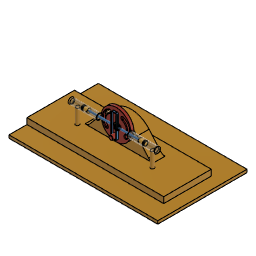
Scotch Yoke Mechanism FINISHED (Autodesk Fusion 360 design; units mm, degrees)
Autodesk Fusion 360 part; units mm, degrees
sketch "Bottom Sketch" plane through (0, 0, 0) normal (0, 0, 1) x (1, 0, 0) in component "Holder"
  line L0 (0, 0) -> (250, 0)
  line L1 (250, 0) -> (250, 150)
  line L2 (250, 150) -> (0, 150)
  line L3 (0, 150) -> (0, 0)
  dimension "d1" = 250
  dimension "d2" = 150
  constraint horizontal L0
  constraint vertical L1
  constraint horizontal L2
  constraint vertical L3
  constraint coincident L0.start L3.end
  measures "d1" distance of L0.start L0.end
  measures "d2" distance of L0.start L2.end
extrude "Extrude1" add sketch "Bottom Sketch" along normal blind 5 makes body 1 in component "Holder"
sketch "holder" plane through (0, 0, 5) normal (0, 0, 1) x (-1, 0, 0) in component "Holder"
  line L0 (0, -150) -> (0, 0)
  line L1 (0, 0) -> (-250, 0)
  line L2 (-250, 0) -> (-250, -150)
  line L3 (-250, -150) -> (0, -150)
  circle A0 centre (-205.8519, -60.5247) radius 10
  line L4 (0, -150) -> (-125, -150)
  line L5 (-125, -150) -> (-125, 0)
  circle A1 centre (-44.1481, -60.5247) radius 10
  dimension "d5" = 20
  dimension "d6" = 125
  constraint coincident L0.start L3.end
  constraint midpoint L3 L4.end
  constraint midpoint L1 L5.end
  constraint symmetric A0 L5 A1
  measures "d5" diameter of A0
  measures "d6" distance of L0.start L4.end
extrude "Extrude2" add sketch "holder" along normal blind 10 separate body contours A0 makes body 2 in component "Holder"
extrude "Extrude3" add sketch "holder" along normal blind 10 contours A1 bodies 1 in component "Holder"
combine "Combine1" operation add target body 1 tool bodies 2 in component "Holder"
sketch "holder nr2" plane through (0, 0, 15) normal (0, 0, 1) x (-1, 0, 0) in component "Holder"
  circle A0 centre (-205.8519, -60.5247) radius 10
  line L0 (-240, -20) -> (-10, -20)
  line L1 (-10, -20) -> (-10, -100)
  line L2 (-10, -100) -> (-240, -100)
  line L3 (-240, -100) -> (-240, -20)
  constraint horizontal L0
  constraint vertical L1
  constraint horizontal L2
  constraint vertical L3
extrude "Extrude4" add sketch "holder nr2" along normal blind 10 contours A0 | L0 L1 L2 L3 bodies 1 in component "Holder"
sketch "holder circle" plane through (0, 100, 0) normal (0, 1, 0) x (-1, 0, 0) in component "Holder"
  line L0 (-240, 15) -> (-10, 15)
  line L1 (-10, 15) -> (-10, 25)
  line L2 (-10, 25) -> (-240, 25)
  line L3 (-240, 25) -> (-240, 15)
  line L4 (-177.5741, 25) -> (-155.4332, 50.958)
  line L5 (-125, 65) -> (-125, 15)
  line L6 (-72.4259, 25) -> (-94.5668, 50.958)
  arc A0 (-94.5668, 50.958) -> (-155.4332, 50.958) centre (-125, 25) ccw
  constraint coincident L2 L4.start
  constraint midpoint L0 L5.end
  constraint symmetric L4.start L5 L6.start
  constraint symmetric L4.end L5 L6.end
extrude "Extrude5" add sketch "holder circle" along normal blind -20 and the other way blind 40 contours L2 L5 L6 A0 | L2 L4 L5 A0 bodies 1 in component "Holder"
sketch "crank" plane through (0, 0, 0) normal (0, 1, 0) x (1, 0, 0) in component "Crank"
  circle A0 centre (125, -55) radius 25
  circle A1 centre (125, -55) radius 3
  circle A2 centre (125, -40) radius 3.5
  dimension "d18" = 50
  dimension "d19" = 6
  dimension "d24" = 7
  constraint concentric A0 A1
  measures "d18" diameter of A0
  measures "d19" diameter of A1
  measures "d24" diameter of A2
extrude "Extrude1'" add sketch "crank" along normal blind 60 and the other way blind -55 separate body contours A0 | A2 makes body 3 in component "Crank"
extrude "Extrude2'" add sketch "crank" along normal blind 60 and the other way blind -46 contours A2 bodies 3 in component "Crank"
fillet "Fillet1" radius 0.5 1 faces at (123.924, 46, 39.8261) on bodies 3 in component "Crank"
sketch "crank holder" plane through (0, 60, 0) normal (0, -1, 0) x (1, 0, 0) in component "Holder"
  line L0 (94.5668, 50.958) -> (72.4259, 25)
  line L1 (72.4259, 25) -> (177.5741, 25)
  line L2 (177.5741, 25) -> (155.4332, 50.958)
  arc A0 (155.4332, 50.958) -> (94.5668, 50.958) centre (125, 25) ccw
  circle A1 centre (125, 55) radius 2.996
extrude "Extrude6" add sketch "crank holder" along normal blind 6 contours A1 bodies 1 in component "Holder"
fillet "Fillet1'" radius 0.25 1 edges at (122.2068, 54, 53.9166) on bodies 1 in component "Holder"
sketch "crank button" plane through (0, 54, 0) normal (0, -1, 0) x (1, 0, 0) in component "Holder"
  circle A0 centre (125, 55) radius 2.746
  circle A1 centre (125, 55) radius 1.0708
  constraint concentric A0 A1
extrude "Extrude7" add sketch "crank button" along normal blind 0.5 contours A1 bodies 1 in component "Holder"
fillet "Fillet2" radius 0.5 1 edges at (124.0017, 53.5, 54.6128) on bodies 1 in component "Holder"
sketch "crank design" plane through (0, 55, 0) normal (0, -1, 0) x (1, 0, 0) in component "Crank"
  circle A0 centre (125, 40) radius 3.5
  circle A1 centre (125, 55) radius 3
  circle A2 centre (125, 55) radius 25
  line L0 (125, 58) -> (125, 30)
  arc A3 (139.6103, 45.9052) -> (135.2122, 67.1617) centre (130, 55) ccw
  arc A4 (142.5156, 43.1557) -> (136.7878, 70.8383) centre (130, 55) ccw
  arc A5 (113.2122, 70.8383) -> (107.4844, 43.1557) centre (120, 55) ccw
  arc A6 (114.7878, 67.1617) -> (110.3897, 45.9052) centre (120, 55) ccw
  arc A7 (136.7878, 70.8383) -> (135.2122, 67.1617) centre (136, 69) ccw
  arc A8 (139.6103, 45.9052) -> (142.5156, 43.1557) centre (141.0629, 44.5304) ccw
  arc A9 (107.4844, 43.1557) -> (110.3897, 45.9052) centre (108.9371, 44.5304) ccw
  arc A10 (114.7878, 67.1617) -> (113.2122, 70.8383) centre (114, 69) ccw
  constraint coincident A2 L0.end
  constraint vertical L0
  constraint symmetric L0 A7 A10
  constraint symmetric L0 A8 A9
  constraint symmetric L0 A4.end A5.start
  constraint symmetric L0 A3.end A6.start
  constraint symmetric L0 A3.start A6.end
  constraint symmetric L0 A3 A6
  constraint symmetric L0 A4 A5
  constraint symmetric L0 A4.start A5.end
  constraint coincident A1 L0.start
extrude "Extrude3'" cut sketch "crank design" against normal blind 5 contours A3 A4 A7 A8 | A5 A6 A9 A10 bodies 3 in component "Crank"
fillet "Fillet2'" radius 1 tangency weight 1.30642 8 edges at (139.6882, 55, 43.0778) (142.9571, 55, 57.6809) (134.1617, 55, 69.7878) (146.8741, 55, 58.4914) (115.8383, 55, 69.7878) (107.0429, 55, 57.6809) (110.3118, 55, 43.0778) (103.1259, 55, 58.4914) on bodies 3 in component "Crank"
fillet "Fillet3" radius 1 8 edges at (142.9571, 60, 57.6809) (139.6882, 60, 43.0778) (146.8741, 60, 58.4914) (134.1617, 60, 69.7878) (110.3118, 60, 43.0778) (107.0429, 60, 57.6809) (115.8383, 60, 69.7878) (103.1259, 60, 58.4914) on bodies 3 in component "Crank"
fillet "Fillet3'" radius 10 2 edges at (72.4259, 70, 25) (177.5741, 70, 25) on bodies 1 in component "Holder"
sketch "slider part" plane through (0, 55, 0) normal (0, -1, 0) x (1, 0, 0) in component "Slider"
  spline S0 degree 3 poles (138.884, 46.5925) (138.6466, 46.3416) (138.4537, 46.0504) (138.0969, 45.2368) (138.0174, 44.6763) (138.144, 43.7208) (138.2876, 43.3168) (138.644, 42.7368) (138.8105, 42.5316) (139.0008, 42.3515) (139.2187, 42.1453) (139.4677, 41.9721) (140.1668, 41.6275) (140.6495, 41.5207) (141.7193, 41.5441) (142.3066, 41.7372) (142.9525, 42.1918) (143.1044, 42.3231) (143.2419, 42.4684) knots -0.939789 -0.939789 -0.939789 -0.939789 -0.836626 -0.836626 -0.673634 -0.673634 -0.548256 -0.548256 -0.469895 -0.469895 -0.469895 -0.380181 -0.380181 -0.236639 -0.236639 -0.059698 -0.059698 0 0 0 0
  spline S1 degree 3 poles (134.8182, 66.2426) (135.4369, 65.9774) (136.0273, 65.6646) (138.0714, 64.3564) (139.3378, 63.092) (141.1843, 60.2232) (141.7952, 58.6395) (142.2944, 55.6272) (142.2853, 54.2147) (141.8379, 51.7146) (141.474, 50.6097) (140.4268, 48.4906) (139.7247, 47.4809) (138.884, 46.5925) knots -3.290631 -3.290631 -3.290631 -3.290631 -3.089591 -3.089591 -2.564742 -2.564742 -2.06659 -2.06659 -1.649506 -1.649506 -1.305101 -1.305101 -0.939789 -0.939789 -0.939789 -0.939789
  spline S2 degree 3 poles (137.1818, 71.7574) (136.4622, 72.0658) (135.6228, 72.0768) (134.3103, 71.5579) (133.7994, 71.1345) (133.1483, 70.102) (132.9855, 69.5098) (133.0133, 68.4575) (133.1348, 67.9974) (133.5483, 67.2219) (133.8226, 66.895) (134.3532, 66.479) (134.5789, 66.3451) (134.8182, 66.2426) knots -4.230421 -4.230421 -4.230421 -4.230421 -3.996672 -3.996672 -3.807702 -3.807702 -3.631502 -3.631502 -3.492839 -3.492839 -3.368403 -3.368403 -3.290631 -3.290631 -3.290631 -3.290631
  spline S3 degree 3 poles (143.2419, 42.4684) (143.9145, 43.1791) (144.5233, 43.9358) (146.1358, 46.3053) (146.9521, 48.03) (148.237, 52.385) (148.4232, 55.0933) (147.6191, 60.4311) (146.5868, 63.0502) (144.1198, 66.6461) (143.0272, 67.8564) (140.4122, 70.0755) (138.8575, 71.0393) (137.1818, 71.7574) knots -7.734434 -7.734434 -7.734434 -7.734434 -7.44224 -7.44224 -6.876501 -6.876501 -6.081666 -6.081666 -5.25889 -5.25889 -4.774784 -4.774784 -4.230421 -4.230421 -4.230421 -4.230421
  circle A0 centre (125, 40) radius 3.5
  circle A1 centre (125, 55) radius 3
  circle A2 centre (125, 55) radius 25
  spline S4 degree 3 poles (115.1818, 66.2426) (115.4992, 66.3786) (115.7918, 66.5694) (116.4422, 67.1747) (116.7376, 67.6575) (117.0005, 68.5848) (117.0291, 69.0127) (116.9321, 69.6865) (116.8607, 69.9409) (116.7574, 70.1818) (116.6393, 70.4575) (116.4795, 70.7152) (115.9745, 71.309) (115.5739, 71.5986) (114.5826, 72.0016) (113.9669, 72.0574) (113.1936, 71.8965) (113.002, 71.8362) (112.8182, 71.7574) knots -0.939789 -0.939789 -0.939789 -0.939789 -0.836626 -0.836626 -0.673634 -0.673634 -0.548256 -0.548256 -0.469895 -0.469895 -0.469895 -0.380181 -0.380181 -0.236639 -0.236639 -0.059698 -0.059698 0 0 0 0
  spline S5 degree 3 poles (111.116, 46.5925) (110.6533, 47.0814) (110.2356, 47.6028) (108.8785, 49.6147) (108.2178, 51.2779) (107.6613, 54.6439) (107.729, 56.3399) (108.4661, 59.303) (109.035, 60.5959) (110.4378, 62.7133) (111.2103, 63.583) (113.0124, 65.1126) (114.0575, 65.7607) (115.1818, 66.2426) knots -3.290631 -3.290631 -3.290631 -3.290631 -3.089591 -3.089591 -2.564742 -2.564742 -2.06659 -2.06659 -1.649506 -1.649506 -1.305101 -1.305101 -0.939789 -0.939789 -0.939789 -0.939789
  spline S6 degree 3 poles (106.7581, 42.4684) (107.2962, 41.8998) (108.0624, 41.5566) (109.473, 41.512) (110.11, 41.6979) (111.1173, 42.3872) (111.5017, 42.8663) (111.8939, 43.8432) (111.9649, 44.3138) (111.8931, 45.1896) (111.771, 45.5986) (111.449, 46.1909) (111.295, 46.4034) (111.116, 46.5925) knots -4.230421 -4.230421 -4.230421 -4.230421 -3.996672 -3.996672 -3.807702 -3.807702 -3.631502 -3.631502 -3.492839 -3.492839 -3.368403 -3.368403 -3.290631 -3.290631 -3.290631 -3.290631
  spline S7 degree 3 poles (112.8182, 71.7574) (111.9188, 71.3719) (111.0598, 70.919) (108.6393, 69.3839) (107.2056, 68.1247) (104.2981, 64.6372) (103.0524, 62.2252) (101.6724, 57.0066) (101.5806, 54.1928) (102.4181, 49.9132) (102.9406, 48.3687) (104.4603, 45.2941) (105.505, 43.7925) (106.7581, 42.4684) knots -7.734434 -7.734434 -7.734434 -7.734434 -7.44224 -7.44224 -6.876501 -6.876501 -6.081666 -6.081666 -5.25889 -5.25889 -4.774784 -4.774784 -4.230421 -4.230421 -4.230421 -4.230421
  line L0 (128.5, 36.3298) -> (121.347, 36.3298)
  line L1 (121.347, 36.3298) -> (128.6536, 36.3298)
  line L2 (128.6536, 36.3298) -> (128.6536, 73.7122)
  line L3 (128.6536, 73.7122) -> (121.347, 73.7122)
  line L4 (121.347, 73.7122) -> (121.347, 36.3298)
  line L5 (120.0866, 35.0694) -> (129.914, 35.0694)
  line L6 (129.914, 35.0694) -> (129.914, 74.9727)
  line L7 (129.914, 74.9727) -> (120.0866, 74.9727)
  line L8 (120.0866, 74.9727) -> (120.0866, 35.0694)
  dimension "d47" = 1.2604
  constraint horizontal L1
  constraint vertical L2
  constraint horizontal L3
  constraint vertical L4
extrude "Extrude1''" add sketch "slider part" along normal blind 4 separate body contours L5 L6 L7 L8 makes body 4 in component "Slider"
extrude "Extrude2''" cut sketch "slider part" along normal blind 0 and the other way blind -0.8 contours L5 L6 L7 L8 bodies 4 in component "Slider"
fillet "Fillet1''" radius 2 2 edges at (120.0866, 52.6, 74.9727) (129.914, 52.6, 74.9727) on bodies 4 in component "Slider"
fillet "Fillet2''" radius 1.5 2 edges at (120.0866, 52.6, 35.0694) (129.914, 52.6, 35.0694) on bodies 4 in component "Slider"
fillet "Fillet3''" radius 0.5 4 faces at (126.218, 53.1333, 73.7122) (121.347, 53.1333, 61.2514) (128.6536, 53.1333, 48.7906) (123.7825, 53.1333, 36.3298) on bodies 4 in component "Slider"
sketch "slider left+right part" plane through (129.914, 0, 0) normal (1, 0, 0) x (0, 1, 0) in component "Slider"
  line L0 (51, 36.5694) -> (54.2, 36.5694)
  line L1 (54.2, 36.5694) -> (54.2, 72.9727)
  line L2 (54.2, 72.9727) -> (51, 72.9727)
  line L3 (51, 72.9727) -> (51, 36.5694)
  line L4 (52.6, 72.9727) -> (52.6, 54.7727)
  circle A0 centre (52.6, 54.7727) radius 1.5
  dimension "d60" = 18.2
  dimension "d61" = 3
  constraint midpoint L2 L4.start
  constraint perpendicular L0 L4
  constraint coincident L4.end A0.centre
  measures "d60" distance of L4.start L4.end
  measures "d61" diameter of A0
extrude "Extrude3''" add sketch "slider left+right part" along normal blind 40 contours A0 bodies 4 in component "Slider"
extrude "Extrude4'" add sketch "slider left+right part" along normal blind -50 and the other way blind 9 contours A0 bodies 4 in component "Slider"
sketch "piston1&2" plane through (129.914, 0, 0) normal (1, 0, 0) x (0, 1, 0) in component "Pistons"
  circle A0 centre (52.6157, 54.7582) radius 4
  circle A1 centre (52.6157, 54.7582) radius 5
  dimension "d68" = 8
  dimension "d69" = 1
  measures "d68" diameter of A0
extrude "Extrude1'''" add sketch "piston1&2" along normal blind 67 and the other way blind -21 separate body makes body 5 in component "Pistons"
extrude "Extrude2'''" add sketch "piston1&2" along normal blind -31 and the other way blind 78 separate body makes body 6 in component "Pistons"
sketch "piston 1 interior part" plane through (129.914, 0, 0) normal (1, 0, 0) x (0, 1, 0) in component "Pistons"
  circle A0 centre (52.592, 54.7678) radius 3.25
  circle A1 centre (52.592, 54.7678) radius 3.45
  dimension "d86" = 6.5
  dimension "d107" = 0.2
  measures "d86" diameter of A0
extrude "Extrude5'" add sketch "piston 1 interior part" along normal blind 48 and the other way blind -38 separate body contours A0 makes body 7 in component "Pistons"
sketch "piston 1 hole for screw" plane through (0, 0, 0) normal (0, 1, 0) x (1, 0, 0) in component "Pistons"
  circle A0 centre (169, -55) radius 0.5
extrude "Extrude7'" cut sketch "piston 1 hole for screw" along normal blind 51.3 bodies 7 in component "Pistons"
extrude "Extrude8" add sketch "piston 1 interior part" along normal blind -48 and the other way blind 58 separate body contours A0 makes body 8 in component "Pistons"
sketch "piston 2 hole for screw" plane through (0, 0, 0) normal (0, 1, 0) x (1, 0, 0) in component "Pistons"
  circle A0 centre (81, -55) radius 0.5
  dimension "d101" = 1
  measures "d101" diameter of A0
extrude "Extrude6'" cut sketch "piston 2 hole for screw" along normal blind 51.3 bodies 4 in component "Slider"
extrude "Extrude9" cut sketch "piston 2 hole for screw" along normal blind 51.3 bodies 8 in component "Pistons"
extrude "Extrude10" add sketch "piston 1 interior part" along normal blind -58 and the other way blind 57.5 bodies 8 in component "Pistons"
extrude "Extrude11" add sketch "piston 1 interior part" along normal blind -56.7 and the other way blind 57 bodies 8 in component "Pistons"
extrude "Extrude12" add sketch "piston 1 interior part" along normal blind -55.7 and the other way blind 56 bodies 8 in component "Pistons"
extrude "Extrude13" add sketch "piston 1 interior part" along normal blind -48 and the other way blind 55 bodies 8 in component "Pistons"
extrude "Extrude14" cut sketch "piston 2 hole for screw" along normal blind 51.3 bodies 8 in component "Pistons"
extrude "Extrude15" add sketch "piston 1 interior part" along normal blind 48 and the other way blind -47.5 bodies 7 in component "Pistons"
fillet "Fillet1'''" radius 0.25 1 edges at (71.914, 49.3755, 56.0154) on bodies 8 in component "Pistons"
fillet "Fillet2'''" radius 0.25 1 edges at (177.914, 49.3755, 53.5203) on bodies 7 in component "Pistons"
extrude "Extrude16" add sketch "piston 1 interior part" along normal blind 47 and the other way blind -46.7 bodies 7 in component "Pistons"
extrude "Extrude17" add sketch "piston 1 interior part" along normal blind 46 and the other way blind -45.7 bodies 7 in component "Pistons"
extrude "Extrude18" add sketch "piston 1 interior part" along normal blind 45 and the other way blind -38 bodies 7 in component "Pistons"
extrude "Extrude19" cut sketch "piston 1 hole for screw" along normal blind 51.3 bodies 7 in component "Pistons"
extrude "Extrude20" cut 1 faces at (79.914, 53.3169, 54.6981) along direction (-1, 0, 0) blind 2 on bodies 4 bodies 8 in component "Pistons"
extrude "Extrude7''" cut 1 faces at (168.9867, 51.3, 54.8449) along direction (0, -1, 0) blind 2.4 and the other way blind 0.15 on bodies 7 bodies 4 in component "Slider"
extrude "Extrude21" cut 1 faces at (168.9867, 51.3, 54.8449) along direction (0, -1, 0) blind 2.4 and the other way blind 0.15 on bodies 7 bodies 7 in component "Pistons"
copy_body "CutPasteBodies1" bodies 7 8 removing the originals makes body 9 makes body 10 in component "Slider"
delete_face "DeleteFace1" 1 faces at (128.9677, 51.0358, 48.9573) on bodies 4 in component "Slider"
delete_face "DeleteFace2" 1 faces at (121.338, 51.4054, 61.0848) on bodies 4 in component "Slider"
extrude "Extrude22" add sketch "piston1&2" along normal blind -76 and the other way blind 78 contours A0 bodies 6 in component "Pistons"
extrude "Extrude24" add sketch "piston1&2" along normal blind 67 and the other way blind -65 contours A0 bodies 5 in component "Pistons"
sketch "holder for pistons" plane through (0, 0, 25) normal (0, 0, 1) x (-1, 0, 0) in component "Holder"
  line L0 (-182.1881, -60) -> (-67.8119, -60)
  line L1 (-67.8119, -60) -> (-67.8119, -80)
  line L2 (-67.8119, -80) -> (-182.1881, -80)
  line L3 (-182.1881, -80) -> (-182.1881, -60)
  line L4 (-240, -100) -> (-10, -100)
  line L5 (-10, -100) -> (-10, -20)
  line L6 (-10, -20) -> (-240, -20)
  line L7 (-240, -20) -> (-240, -100)
  circle A0 centre (-188, -53) radius 3
  line L8 (-125, -100) -> (-125, 0)
  line L9 (-125, 0) -> (-125, -150)
  circle A1 centre (-62, -53) radius 3
  dimension "d179" = 6
  constraint perpendicular L6 L8
  constraint perpendicular L6 L9
  constraint coincident L4 L8.start
  constraint symmetric A0 L9 A1
  measures "d179" diameter of A0
extrude "Extrude8'" add sketch "holder for pistons" along normal blind 30 contours A0 | A1 bodies 1 in component "Holder"
sketch "sketch for piston holder cut" plane through (196.914, 0, 0) normal (1, 0, 0) x (0, 1, 0) in component "Holder"
  circle A0 centre (52.6157, 54.7582) radius 5
  circle A1 centre (52.6157, 54.7582) radius 5.1
  dimension "d184" = 10.2
  constraint concentric A0 A1
  measures "d184" diameter of A1
extrude "Extrude9'" cut sketch "sketch for piston holder cut" against normal blind 15 contours A0 bodies 1 in component "Holder"
extrude "Extrude10'" cut sketch "sketch for piston holder cut" along normal blind -120 and the other way blind 160 contours A0 bodies 1 in component "Holder"
component "Holder" placed x (1, 0, 0) y (0, 1, 0) z (0, 0, 1) at (0, 0, 0)
component "Crank" placed x (0.967268, 0, -0.253758) y (0, 1, 0) z (0.253758, 0, 0.967268) at (-9.8652, 0, 33.52)
component "Slider" placed x (1, 0, 0) y (0, 1, 0) z (0, 0, 1) at (-3.9584, 0, 0)
component "Pistons" placed x (1, 0, 0) y (0, 1, 0) z (0, 0, 1) at (0, 0, 0)
equation "d60 = ( 36.4 / 2 ) * 1 mm"
named bodies: "bottom holder", "crank body", "SLIDER", "piston 1", "piston 2", "piston 1 interior part", "piston 2 interior part"
